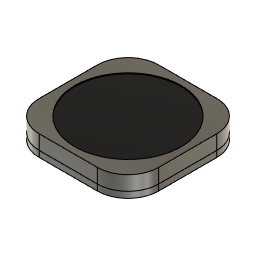
Cirque Holder Flat v12 (Autodesk Fusion 360 design; units mm, degrees)
Autodesk Fusion 360 part; units mm, degrees
note: some values were not read from the file. Chosen so that the rebuilt part matches the saved one: a side; which face or edge a step refers to. Set by a fixed rule: which sketch regions a step uses.
sketch "Sketch1" plane through (0, 0, 0) normal (0, 0, 1) x (1, 0, 0)
  circle A0 centre (0, 0) radius 17.75
  circle A1 centre (0, 0) radius 17.5
  line L0 (9.5, -19.5) -> (-9.5, -19.5)
  line L1 (-19.5, -9.5) -> (-19.5, 9.5)
  line L2 (-9.5, 19.5) -> (9.5, 19.5)
  line L3 (19.5, 9.5) -> (19.5, -9.5)
  line L4 (19.5, -19.5) -> (-19.5, 19.5) construction
  line L5 (-19.5, -19.5) -> (19.5, 19.5) construction
  arc A2 (19.5, 9.5) -> (9.5, 19.5) centre (9.5, 9.5) ccw
  arc A3 (9.5, -19.5) -> (19.5, -9.5) centre (9.5, -9.5) ccw
  arc A4 (-19.5, -9.5) -> (-9.5, -19.5) centre (-9.5, -9.5) ccw
  arc A5 (-9.5, 19.5) -> (-19.5, 9.5) centre (-9.5, 9.5) ccw
  circle A6 centre (0, 0) radius 17.35
  line L6 (-12.5052, 12.5052) -> (-16.5711, 12.5052) construction
  line L7 (-16.5711, 12.5052) -> (-16.5711, 16.5711) construction
  line L8 (-16.5711, 16.5711) -> (-12.5052, 16.5711) construction
  line L9 (-12.5052, 16.5711) -> (-12.5052, 12.5052) construction
  line L10 (-12.5052, 16.5711) -> (-16.5711, 12.5052) construction
  circle A7 centre (-14.5381, 14.5381) radius 1.65
  line L11 (0, 0) -> (-17.5, 0) construction
  line L12 (-2.55, -4.6) -> (-19.5, -4.6)
  line L13 (-17.75, -4.6) -> (-17.75, 4.6)
  line L14 (-19.5, 4.6) -> (-2.55, 4.6)
  line L15 (-2.55, 4.6) -> (-2.55, -4.6)
  line L16 (-17.75, 0) -> (-2.55, 0) construction
  circle A8 centre (-14.5381, 14.5381) radius 1.1
  line L17 (-16.7428, -4.55) -> (-19.5, -4.55)
  line L18 (-19.5, -4.55) -> (-19.5, 4.55)
  line L19 (-19.5, 4.55) -> (-16.7428, 4.55)
  line L20 (-17.75, 4.55) -> (-17.75, -4.55)
  line L21 (0, -19.5) -> (0, 19.5) construction
  line L22 (-19.5, 0) -> (19.5, 0) construction
  circle A9 centre (-14.5381, -14.5381) radius 1.65
  circle A10 centre (-14.5381, -14.5381) radius 1.1
  circle A11 centre (14.5381, 14.5381) radius 1.65
  circle A12 centre (14.5381, 14.5381) radius 1.1
  circle A13 centre (14.5381, -14.5381) radius 1.65
  circle A14 centre (14.5381, -14.5381) radius 1.1
  line L23 (-19.5, 0) -> (-17.75, 0) construction
  dimension "d1" = 35.5
  dimension "d2" = 35
  dimension "d7" = 39
  dimension "d8" = 39
  dimension "d9" = 10
  dimension "d16" = 34.7
  dimension "d19" = 3.3
  dimension "d50" = 15.2
  dimension "d51" = 9.2
  dimension "d55" = 2.2
  dimension "d68" = 5.75
  dimension "d78" = 9.1
  constraint coincident A0.centre A1.centre
  constraint concentric A0 A1
  constraint horizontal L0
  constraint perpendicular L0 L1
  constraint parallel L0 L2
  constraint parallel L1 L3
  constraint coincident L4 A0.centre
  constraint coincident L5 A0.centre
  constraint coincident L5.end L2
  constraint coincident L5.end L3
  constraint tangent L2 A2
  constraint tangent L3 A2
  constraint coincident L4.start L0
  constraint coincident L4.start L3
  constraint tangent L0 A3
  constraint tangent L3 A3
  constraint equal A2 A3
  constraint coincident L5.start L1
  constraint coincident L5.start L0
  constraint tangent L1 A4
  constraint tangent L0 A4
  constraint equal A2 A4
  constraint coincident L4.end L1
  constraint coincident L4.end L2
  constraint tangent L1 A5
  constraint tangent L2 A5
  constraint equal A2 A5
  constraint horizontal L6
  constraint vertical L7
  constraint horizontal L8
  constraint vertical L9
  constraint midpoint A5 L7.end
  constraint coincident L4 L6.start
  constraint midpoint L10 A7.centre
  constraint coincident A1 L11.end
  constraint horizontal L11
  constraint horizontal L12
  constraint horizontal L14
  constraint vertical L15
  constraint tangent A0 L13
  constraint midpoint L13 L16.start
  constraint midpoint L15 L16.end
  constraint collinear L11 L16
  constraint concentric A7 A8
  constraint vertical L18
  constraint midpoint L0 L21.start
  constraint midpoint L2 L21.end
  constraint midpoint L1 L22.start
  constraint midpoint L3 L22.end
  constraint symmetric A7 L22 A9
  constraint symmetric A8 L22 A10
  constraint symmetric A7 L21 A11
  constraint symmetric A8 L21 A12
  constraint symmetric L21 A9 A13
  constraint symmetric L21 A10 A14
  constraint collinear L1 L18
  constraint vertical L13
  constraint midpoint L18 L22.start
  constraint midpoint L20 L16.start
  constraint collinear L22 L23
  constraint horizontal L19
  constraint perpendicular L17 L20
  constraint collinear L13 L20
  constraint coincident L1 L14.start
  constraint coincident L13.end L14
  constraint coincident L1 L12.end
  constraint coincident L12 L13.start
  constraint coincident L20.end L17
  constraint coincident L20.start L19
  constraint coincident A6 L17.start
  constraint coincident A6 L19.end
  measures "d1" diameter of A0
  measures "d2" diameter of A1
  measures "d7" distance of L4.end L5.end
  measures "d8" distance of L5.start L4.end
  measures "d9" radius of A2
  measures "d16" diameter of A6
  measures "d19" diameter of A7
  measures "d50" distance of L13.end L14.end
  measures "d51" distance of L12.start L14.end
  measures "d55" diameter of A8
  measures "d68" distance of L6.start L7.end
  measures "d78" distance of L17 L19
extrude "Extrude8" add sketch "Sketch1" against normal blind 2.5 contours A1 A6 L14 L19 | A1 A6 L12 L14 | A1 A6 L12 L17 | A1 A6 L17 L19 | A6 L12 L14 L15 | A6 L12 L14 L15 makes body 1
extrude "Extrude9" add sketch "Sketch1" along normal blind 0.3 separate body contours A0 A1 L12 L14 | A0 L0 L1 L2 L3 A2 A3 A4 A5 L12 L14 | A0 A1 L14 L19 | A0 L13 L14 L19 | A0 L12 L13 L17 | A0 A1 L12 L17 | A0 A1 L17 L19 | A0 L13 L19 L20 | L1 L13 L14 L19 | A1 A6 L14 L19 | A1 A6 L12 L14 | A0 L13 L17 L20 | A1 A6 L12 L17 | L1 L12 L13 L17 | L1 L13 L17 L18 L19 L20 | A1 A6 L17 L19 | A7 | A8 | A9 | A10 | A11 | A12 | A13 | A14 makes body 2
extrude "Extrude10" add sketch "Sketch1" against normal blind 4.4 contours A0 L0 L1 L2 L3 A2 A3 A4 A5 L12 L14 | A0 L13 L14 L19 | A0 L12 L13 L17 | A0 L13 L19 L20 | L1 L13 L14 L19 | A0 L13 L17 L20 | L1 L12 L13 L17 | L1 L13 L17 L18 L19 L20 | A7 | A8 | A9 | A10 | A11 | A12 | A13 | A14 bodies 2
extrude "Extrude11" cut sketch "Sketch1" along normal blind 2.7 from surface at -4.4 contours A7 | A8 | A9 | A10 | A11 | A12 | A13 | A14 bodies 2
extrude "Extrude12" add sketch "Sketch1" against normal blind 2 from surface at -4.4 separate body contours A0 A1 L12 L14 | A0 L0 L1 L2 L3 A2 A3 A4 A5 L12 L14 | A0 A1 L14 L19 | A0 L13 L14 L19 | A0 L12 L13 L17 | A0 A1 L12 L17 | A0 A1 L17 L19 | A0 L13 L19 L20 | L1 L13 L14 L19 | A1 A6 L14 L19 | A1 A6 L12 L14 | A0 L13 L17 L20 | A1 A6 L12 L17 | L1 L12 L13 L17 | L1 L13 L17 L18 L19 L20 | A1 A6 L17 L19 | A6 L12 L14 L15 | A6 L12 L14 L15 | A7 | A8 | A9 | A10 | A11 | A12 | A13 | A14 makes body 3
extrude "Extrude13" add sketch "Sketch1" along normal up to surface (1.8 mm away) from surface at -4.4 contours A0 A1 L17 L19 | A0 L13 L19 L20 | A0 L13 L17 L20 | L1 L13 L17 L18 L19 L20 | A1 A6 L17 L19 bodies 3
extrude "Extrude14" cut sketch "Sketch1" against normal up to surface (3.8 mm away) from surface at -2.6 contours A6 L12 L14 L15 picked at (-7.4833, 0) bodies 3
extrude "Extrude15" cut sketch "Sketch1" against normal up to surface (2 mm away) from surface at -4.4 contours A8 | A10 | A12 | A14 bodies 3
extrude "Extrude17" cut sketch "Sketch1" along normal up to surface (1.9 mm away) from surface at -4.4 contours A0 L13 L14 L19 | A0 L12 L13 L17 | A0 L13 L19 L20 | L1 L13 L14 L19 | A0 L13 L17 L20 | L1 L12 L13 L17 | L1 L13 L17 L18 L19 L20 bodies 2
copy_body "Body->Comp1" bodies 2 removing the originals makes body 4 in component "Component"
copy_body "Body->Comp2" bodies 3 removing the originals makes body 5 in component "Component'"
copy_body "Body->Comp3" bodies 1 removing the originals makes body 6 in component "Component''"
component "Component" placed x (1, 0, 0) y (0, 1, 0) z (0, 0, 1) at (0, 0, 0)
component "Component'" placed x (1, 0, 0) y (0, 1, 0) z (0, 0, 1) at (0, 0, 0)
component "Component''" placed x (1, 0, 0) y (0, 1, 0) z (0, 0, 1) at (0, 0, 0)
equation "d1 = size_dia + 0.5 mm"
equation "d2 = size_dia"
equation "d7 = size_dia + padding"
equation "d8 = size_dia + padding"
equation "d9 = corner_radius"
equation "d16 = size_dia - lip"
equation "d19 = hole_dia"
equation "hole_dia = 3.3 mm"
equation "notch_width = 9.2 mm"
equation "notch_depth = 15.2 mm"
equation "d50 = notch_depth"
equation "d51 = notch_width"
equation "d68 = hole_offset"
equation "size_dia = 35 mm"
equation "lip = 0.3 mm"
equation "depth = 6 mm"
equation "padding = 4 mm"
equation "hole_offset = 5.75 mm"
equation "corner_radius = 10 mm"
equation "d78 = notch_width - 0.1 mm"
